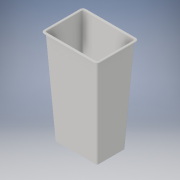
# Autodesk Inventor part: recycle and trash bin
Saved by Autodesk Inventor 2017 (Build 210142000, 142)
## iProperties
Created: 2018-03-26
Part Number: recycle and trash bin
Material: Generic
Document SubType Name: Modeling
Designer: Braxton
Density: 1 g/cm^3
Appearance: Default
Author: Braxton
Autodesk Inventor part; units mm, degrees
ref_plane "YZ Plane" through (0, 0, 0) normal (1, 0, 0) x (0, 1, 0)
ref_plane "XY Plane" through (0, 0, 0) normal (0, 0, 1) x (1, 0, 0)
sketch "Sketch1" plane through (0, 0, 0) normal (0, 1, 0) x (-1, 0, 0)
  line L0 (17.8888, -12.7) -> (0, -12.7)
  line L1 (0, 12.7) -> (17.8888, 12.7)
  line L2 (19.05, 11.5388) -> (19.05, -11.5388)
  arc A0 (17.8888, -12.7) -> (19.05, -11.5388) centre (17.8888, -11.5388) ccw
  line L3 (0, -12.7) -> (0, 12.7) construction
  arc A1 (19.05, 11.5388) -> (17.8888, 12.7) centre (17.8888, 11.5388) ccw
  line L4 (17.8888, -12.4629) -> (0, -12.4629)
  line L5 (0, 12.4629) -> (17.8888, 12.4629)
  line L6 (18.8129, 11.5388) -> (18.8129, -11.5388)
  arc A2 (17.8888, -12.4629) -> (18.8129, -11.5388) centre (17.8888, -11.5388) ccw
  arc A3 (18.8129, 11.5388) -> (17.8888, 12.4629) centre (17.8888, 11.5388) ccw
  line L7 (-17.8888, -12.7) -> (0, -12.7)
  line L8 (0, 12.7) -> (-17.8888, 12.7)
  line L9 (-19.05, 11.5388) -> (-19.05, -11.5388)
  arc A4 (-19.05, -11.5388) -> (-17.8888, -12.7) centre (-17.8888, -11.5388) ccw
  arc A5 (-17.8888, 12.7) -> (-19.05, 11.5388) centre (-17.8888, 11.5388) ccw
  line L10 (-17.8888, -12.4629) -> (0, -12.4629)
  line L11 (0, 12.4629) -> (-17.8888, 12.4629)
  line L12 (-18.8129, 11.5388) -> (-18.8129, -11.5388)
  arc A6 (-18.8129, -11.5388) -> (-17.8888, -12.4629) centre (-17.8888, -11.5388) ccw
  arc A7 (-17.8888, 12.4629) -> (-18.8129, 11.5388) centre (-17.8888, 11.5388) ccw
  point P0 (0, 0)
  point P1 (0, 0)
  dimension "d2" = 0.2371
  dimension "d3" = 0.2371
  dimension "d4" = 0.2371
  dimension "d6" = 19.05
  dimension "d7" = 25.4
  dimension "d17" = 0.9241
  constraints: 26 end point, 16 point on circle, 12 symmetric about line, 8 centre point, 6 tangent, 2 concentric, 2 horizontal, 2 parallel, 1 coincident, 1 equal radius, 1 midpoint, 1 point on line, 4 other
  measures "d2" distance between parallel lines of L0 L4
  measures "d3" distance between parallel lines of L1 L5
  measures "d4" distance between parallel lines of L2 L6
  measures "d6" distance between parallel lines of L2 L3
  measures "d7" distance between parallel lines of L1 L0
  measures "d17" radius of A2
extrude "bottom of bin" add sketch "Sketch1" against normal blind 0.2371 contours L0 L7 A4 L9 A5 L8 L1 A1 L2 A0 | L4 L10 A6 L12 A7 L11 L5 A3 L6 A2
ref_plane "Work Plane1" through (0, 84.6667, 0) normal (0, 1, 0) x (-1, 0, 0)
sketch "Sketch2" plane through (0, 84.6667, 0) normal (0, 1, 0) x (-1, 0, 0)
  line L0 (0, -16.9333) -> (22.3592, -16.9333)
  line L1 (23.2833, -16.0092) -> (23.2833, 16.0092)
  line L2 (22.3592, 16.9333) -> (0, 16.9333)
  line L3 (17.8888, -12.7) -> (-17.8888, -12.7) projected
  line L4 (17.8888, 12.7) -> (-17.8888, 12.7) projected
  line L5 (19.05, -11.5388) -> (19.05, 11.5388) projected
  line L6 (0, -17.1704) -> (22.3592, -17.1704)
  line L7 (23.5204, -16.0092) -> (23.5204, 16.0092)
  line L8 (22.3592, 17.1704) -> (0, 17.1704)
  arc A0 (22.3592, -16.9333) -> (23.2833, -16.0092) centre (22.3592, -16.0092) ccw
  arc A1 (23.2833, 16.0092) -> (22.3592, 16.9333) centre (22.3592, 16.0092) ccw
  arc A2 (23.5204, 16.0092) -> (22.3592, 17.1704) centre (22.3592, 16.0092) ccw
  arc A3 (22.3592, -17.1704) -> (23.5204, -16.0092) centre (22.3592, -16.0092) ccw
  line L9 (0, -8.1161) -> (0, 0) construction
  line L10 (0, -16.9333) -> (-22.3592, -16.9333)
  line L11 (-23.2833, -16.0092) -> (-23.2833, 16.0092)
  line L12 (-22.3592, 16.9333) -> (0, 16.9333)
  line L13 (0, -17.1704) -> (-22.3592, -17.1704)
  line L14 (-23.5204, -16.0092) -> (-23.5204, 16.0092)
  line L15 (-22.3592, 17.1704) -> (0, 17.1704)
  arc A4 (-23.2833, -16.0092) -> (-22.3592, -16.9333) centre (-22.3592, -16.0092) ccw
  arc A5 (-22.3592, 16.9333) -> (-23.2833, 16.0092) centre (-22.3592, 16.0092) ccw
  arc A6 (-22.3592, 17.1704) -> (-23.5204, 16.0092) centre (-22.3592, 16.0092) ccw
  arc A7 (-23.5204, -16.0092) -> (-22.3592, -17.1704) centre (-22.3592, -16.0092) ccw
  point P0 (0, 0)
  dimension "d11" = 4.2333
  dimension "d12" = 4.2333
  dimension "d13" = 4.2333
  dimension "d14" = 0.2371
  dimension "d15" = 0.2371
  dimension "d16" = 0.2371
  dimension "d18" = 0.9241
  dimension "d19" = 0.9241
  constraints: 26 end point, 16 point on circle, 12 symmetric about line, 8 centre point, 6 tangent, 2 concentric, 2 horizontal, 2 parallel, 2 perpendicular, 1 coincident, 1 vertical, 4 other
  measures "d11" distance between parallel lines of L3 L0
  measures "d12" distance between parallel lines of L4 L2
  measures "d13" distance between parallel lines of L5 L1
  measures "d14" distance between parallel lines of L6 L0
  measures "d15" distance between parallel lines of L7 L1
  measures "d16" distance between parallel lines of L2 L8
  measures "d18" radius of A0
  measures "d19" radius of A1
loft "loft make" add profiles "Sketch2", "Sketch1" contours L10 A4 L11 A5 L12 L2 A1 L1 A0 L0 | L13 A7 L14 A6 L15 L8 A2 L7 A3 L6 / L0 L7 A4 L9 A5 L8 L1 A1 L2 A0 | L4 L10 A6 L12 A7 L11 L5 A3 L6 A2
loft "loft cut" cut profiles "Sketch2", "Sketch1" contours L10 A4 L11 A5 L12 L2 A1 L1 A0 L0 / L4 L10 A6 L12 A7 L11 L5 A3 L6 A2
sketch "Sketch3" plane through (0, 0, 0) normal (1, 0, 0) x (0, 1, 0)
  line L0 (84.6667, 16.9333) -> (0, 12.4629) projected
  arc A0 (84.6667, 16.9333) -> (85.3017, 17.6027) centre (84.6313, 17.6027) ccw
  line L1 (85.3017, 17.6027) -> (85.3017, 18.415)
  arc A1 (84.6667, 17.1704) -> (85.0651, 17.6027) centre (84.6313, 17.6027) ccw
  arc A2 (85.3017, 18.415) -> (84.6667, 19.05) centre (84.6667, 18.415) ccw
  line L2 (84.6667, 19.05) -> (84.533, 19.05) construction
  line L3 (84.6667, 19.05) -> (84.6667, 18.8134)
  line L4 (85.0651, 17.6027) -> (85.0651, 18.415)
  arc A3 (85.0651, 18.415) -> (84.6667, 18.8134) centre (84.6667, 18.415) ccw
  line L5 (84.6667, 17.1704) -> (84.6667, 16.0092) projected
  line L6 (84.6667, 16.9333) -> (84.6667, 17.1704)
  point P0 (0, 0)
  dimension "d28" = 2.1167
  dimension "d29" = 0.635
  constraints: 10 end point, 8 point on circle, 6 tangent, 4 centre point, 3 vertical, 2 collinear, 2 concentric, 1 horizontal
  measures "d28" distance of L2.start L0.start
  measures "d29" distance between parallel lines of L3 L1
sweep "lip rim" add profiles "Sketch3" path "Sketch2" path curves L8 A2 L7 A3 L6 L13 A7 L14 A6 L15
equation "\"d3\" = d2"
equation "\"d4\" = d2"
equation "\"d8\" = d2"
equation "\"d12\" = d11"
equation "\"d13\" = d11"
equation "\"d14\" = d2"
equation "\"d15\" = d2"
equation "\"d16\" = d2"
equation "\"d18\" = d17"
equation "\"d19\" = d17"
body "Solid1"
